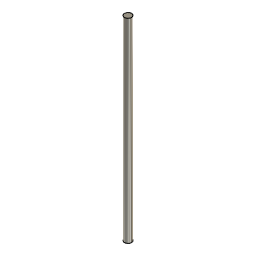
Base_Assemble (Autodesk Fusion 360 archive; units mm, degrees)
design "Rod"
Autodesk Fusion 360 part; units mm, degrees
(part 1 of 2)
sketch "Sketch1" plane through (0, 0, 0) normal (0, 0, 1) x (1, 0, 0)
  circle A0 centre (0, 0) radius 2
  dimension "d1" = 4
  constraint coincident A0.centre origin
  measures "d1" diameter of A0
extrude "Extrude1" add sketch "Sketch1" along normal blind 110

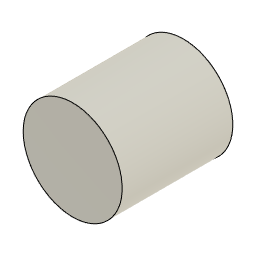
design "_Mug"
Autodesk Fusion 360 part; units mm, degrees
sketch "Sketch1" plane through (0, 0, 0) normal (0, 1, 0) x (1, 0, 0)
  circle A0 centre (0, 0) radius 42.5
  dimension "d1" = 85
  constraint coincident A0.centre origin
  measures "d1" diameter of A0
extrude "Extrude1" add sketch "Sketch1" against normal blind 95

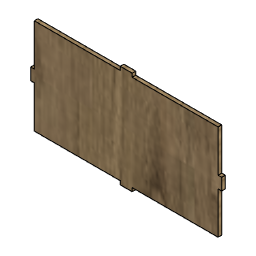
design "LongWall_"
Autodesk Fusion 360 part; units mm, degrees
sketch "Sketch1" plane through (0, 0, 0) normal (0, 1, 0) x (1, 0, 0)
  line L0 (117, 83.2352) -> (40, 83.2352)
  line L1 (40, 83.2352) -> (45, 83.2352)
  line L2 (40, 83.2352) -> (40, 43.2352)
  line L3 (40, 3.2352) -> (45, 3.2352)
  line L4 (117, 43.2352) -> (117, 83.2352)
  line L5 (117, 38.2352) -> (117, 43.2352)
  line L6 (45, 83.2352) -> (45, 86.2352)
  line L7 (120, 83.4704) -> (45, 83.4704)
  line L8 (-37, 83.2352) -> (40, 83.2352)
  line L9 (-37, 3.2352) -> (40, 3.2352)
  line L10 (40, 43.2352) -> (-37, 43.2352)
  line L11 (40, 43.2352) -> (117, 43.2352)
  line L12 (117, 3.2352) -> (40, 3.2352)
  line L13 (45, 0.2352) -> (40, 0.2352)
  line L14 (40, 86.2352) -> (40, 83.2352)
  line L15 (40, 83.2352) -> (40, 43.2352)
  line L16 (117, 43.2352) -> (117, 3.2352)
  line L17 (45, 86.4704) -> (120, 86.4704)
  line L18 (45, 0) -> (120, 0)
  line L19 (120, 48.2352) -> (117, 48.2352)
  line L20 (117, 43.2352) -> (120, 43.2352)
  line L21 (45, 3.2352) -> (45, 0.2352)
  line L22 (120, 43.2352) -> (120, 48.2352)
  line L23 (45, 86.2352) -> (40, 86.2352)
  line L24 (40, 86.2352) -> (40, 83.2352)
  line L25 (120, 0) -> (120, 3)
  line L26 (117, 43.2352) -> (120, 43.2352)
  line L27 (120, 38.2352) -> (117, 38.2352)
  line L28 (40, 43.2352) -> (117, 43.2352)
  line L29 (120, 43.2352) -> (120, 38.2352)
  line L30 (40, 43.2352) -> (-37, 43.2352)
  line L31 (40, 3.2352) -> (40, 43.2352)
  line L32 (117, 48.2352) -> (117, 43.2352)
  line L33 (45, 83.4704) -> (45, 86.4704)
  line L34 (120, 86.4704) -> (120, 83.4704)
  line L35 (45, 3) -> (45, 0)
  line L36 (-40, 48.2352) -> (-37, 48.2352)
  line L37 (-40, 38.2352) -> (-37, 38.2352)
  line L38 (35, 83.2352) -> (35, 86.2352)
  line L39 (40, 3.2352) -> (40, 43.2352)
  line L40 (-40, 43.2352) -> (-40, 48.2352)
  line L41 (40, 0.2352) -> (40, 3.2352)
  line L42 (-40, 43.2352) -> (-40, 38.2352)
  line L43 (35, 83.4704) -> (35, 86.4704)
  line L44 (35, 3.2352) -> (35, 0.2352)
  line L45 (35, 86.4704) -> (-40, 86.4704)
  line L46 (-37, 38.2352) -> (-37, 43.2352)
  line L47 (-37, 43.2352) -> (-37, 3.2352)
  line L48 (40, 3.2352) -> (35, 3.2352)
  line L49 (-37, 43.2352) -> (-37, 83.2352)
  line L50 (120, 3) -> (45, 3)
  line L51 (-40, 83.4704) -> (35, 83.4704)
  line L52 (35, 86.2352) -> (40, 86.2352)
  line L53 (40, 83.2352) -> (35, 83.2352)
  line L54 (-37, 43.2352) -> (-40, 43.2352)
  line L55 (40, 0.2352) -> (40, 3.2352)
  line L56 (-37, 48.2352) -> (-37, 43.2352)
  line L57 (35, 0.2352) -> (40, 0.2352)
  line L58 (-40, 3) -> (35, 3)
  line L59 (-37, 43.2352) -> (-40, 43.2352)
  line L60 (35, 0) -> (-40, 0)
  line L61 (35, 3) -> (35, 0)
  point P0 (0, 86.4704)
  point P1 (80, 86.4704)
  point P2 (80, 0)
  dimension "d1" = 77
  dimension "d2" = 40
  dimension "d3" = 5
  dimension "d4" = 3
  dimension "d5" = 3
  dimension "d6" = 5
  constraint horizontal L9
  constraint vertical L39
  constraint horizontal L10
  constraint vertical L47
  constraint horizontal L48
  constraint vertical L44
  constraint horizontal L57
  constraint vertical L41
  constraint vertical L42
  constraint perpendicular L42 L59
  constraint horizontal L37
  constraint parallel L42 L46
  constraint symmetric P2 origin L39
  constraint symmetric L60.start L18.start L39
  constraint symmetric L60.end L18.end L39
  constraint symmetric L58.start L25.end L39
  constraint symmetric L58.end L35.start L39
  constraint symmetric L9.start L12.start L39
  constraint symmetric L3.start L9.end L39
  constraint symmetric L2.end L10.start L39
  constraint symmetric L4.start L10.end L39
  constraint symmetric L3.end L44.start L39
  constraint symmetric L13.start L44.end L39
  constraint symmetric L13.end L41.start L39
  constraint symmetric L20.end L40.start L39
  constraint symmetric L27.start L37.start L39
  constraint symmetric L5.start L37.end L39
  constraint symmetric P0 origin L28
  constraint symmetric L17.start L18.start L28
  constraint symmetric L17.end L18.end L28
  constraint symmetric L7.start L25.end L28
  constraint symmetric L7.end L35.start L28
  constraint symmetric L9.start L8.start L28
  constraint symmetric L3.start L0.end L28
  constraint symmetric L2.end L10.start L28
  constraint symmetric L10.end L30.end L28
  constraint symmetric L44.start L38.start L28
  constraint symmetric L44.end L38.end L28
  constraint symmetric L13.end L14.start L28
  constraint symmetric L40.start L42.start L28
  constraint symmetric L37.start L36.start L28
  constraint symmetric L37.end L36.end L28
  constraint symmetric L20.end L22.start L28
  constraint symmetric L3.end L1.end L28
  constraint symmetric L5.start L19.end L28
  constraint symmetric L13.start L6.end L28
  constraint symmetric L27.start L19.start L28
  constraint symmetric L4.start L5.end L28
  constraint symmetric L0.end L3.start L28
  constraint symmetric L0.start L12.start L28
  constraint symmetric L43.start L58.end L28
  constraint symmetric L43.end L60.start L28
  constraint symmetric P1 P2 L28
  constraint symmetric L51.start L58.start L28
  constraint symmetric L45.end L60.end L28
  measures "d1" distance of L3.start L9.start
  measures "d2" distance of L10.end L9.start
  measures "d3" distance of L44.start L3.start
  measures "d4" distance of L13.end L3.start
  measures "d5" distance of L10.end L40.start
  measures "d6" distance of L10.end L37.end
extrude "Extrude1" add sketch "Sketch1" along normal blind 3 contours L0 L1 L2 L4 L11 L15 L28 L32 | L0 L1 L6 L14 L23 L24 L33 | L4 L19 L20 L22 L26 L32 | L2 L8 L10 L15 L30 L49 L53 L56 | L8 L14 L24 L38 L43 L52 L53 | L5 L16 L20 L26 L27 L29 | L3 L5 L11 L12 L16 L28 L31 L39 | L9 L10 L30 L31 L39 L46 L47 L48 | L36 L40 L49 L54 L56 L59 | L37 L42 L46 L47 L54 L59 | L9 L41 L44 L48 L55 L57 L61 | L3 L12 L13 L21 L35 L41 L55
ref_plane "WorkPlane1" through (40, 0, -43.2352) normal (0, -1, 0) x (-1, 0, 0)
sketch "Sketch2" plane through (0, 0, 0) normal (0, -1, 0) x (-1, 0, 0)
  line L0 (40, 3.2352) -> (45, 3.2352)
  line L1 (117, 48.2352) -> (117, 43.2352)
  line L2 (35, 83.4704) -> (35, 86.4704)
  line L3 (-37, 43.2352) -> (-37, 83.2352)
  line L4 (120, 48.2352) -> (117, 48.2352)
  line L5 (-37, 43.2352) -> (-37, 3.2352)
  line L6 (-37, 48.2352) -> (-37, 43.2352)
  line L7 (35, 83.2352) -> (35, 86.2352)
  line L8 (35, 3.2352) -> (35, 0.2352)
  line L9 (-40, 48.2352) -> (-37, 48.2352)
  line L10 (35, 3) -> (35, 0)
  line L11 (45, 83.4704) -> (45, 86.4704)
  line L12 (-40, 43.2352) -> (-40, 38.2352)
  line L13 (-40, 3) -> (35, 3)
  line L14 (117, 83.2352) -> (40, 83.2352)
  line L15 (35, 86.2352) -> (40, 86.2352)
  line L16 (117, 3.2352) -> (40, 3.2352)
  line L17 (40, 3.2352) -> (35, 3.2352)
  line L18 (35, 0.2352) -> (40, 0.2352)
  line L19 (-37, 83.2352) -> (40, 83.2352)
  line L20 (40, 83.2352) -> (45, 83.2352)
  line L21 (45, 0.2352) -> (40, 0.2352)
  line L22 (45, 86.2352) -> (40, 86.2352)
  line L23 (120, 43.2352) -> (120, 38.2352)
  line L24 (120, 38.2352) -> (117, 38.2352)
  line L25 (117, 43.2352) -> (117, 83.2352)
  line L26 (-37, 3.2352) -> (40, 3.2352)
  line L27 (-40, 43.2352) -> (-40, 48.2352)
  line L28 (120, 86.4704) -> (120, 83.4704)
  line L29 (45, 83.2352) -> (45, 86.2352)
  line L30 (117, 43.2352) -> (117, 3.2352)
  line L31 (45, 3) -> (45, 0)
  line L32 (45, 3.2352) -> (45, 0.2352)
  line L33 (120, 43.2352) -> (120, 48.2352)
  line L34 (-40, 38.2352) -> (-37, 38.2352)
  line L35 (117, 38.2352) -> (117, 43.2352)
  point P0 (0, 86.4704)
  point P1 (80, 86.4704)
  point P2 (80, 0)
  dimension "d10" = 77
  dimension "d11" = 40
  dimension "d12" = 5
  dimension "d13" = 3
  dimension "d14" = 3
  dimension "d15" = 5
  constraint horizontal L26
  constraint vertical L5
  constraint horizontal L17
  constraint vertical L8
  constraint horizontal L18
  constraint vertical L12
  constraint horizontal L34
  measures "d10" distance of L0.start L5.end
  measures "d11" distance of L3.start L5.end
  measures "d12" distance of L8.start L0.start
  measures "d13" distance of L18.end L0.start
  measures "d14" distance of L12.start L3.start
  measures "d15" distance of L3.start L34.end

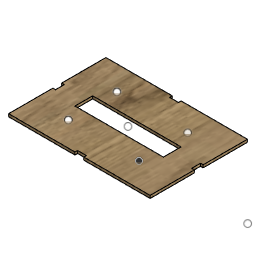
design "Roof"
Autodesk Fusion 360 part; units mm, degrees
sketch "Sketch1" plane through (0, 0, 0) normal (0, 0, 1) x (1, 0, 0)
  line L0 (-162.8452, 27.5) -> (-242.8452, 82.5) construction
  line L1 (-242.8452, 27.5) -> (-239.8452, 27.5)
  line L2 (-162.8452, 82.5) -> (-242.8452, 82.5)
  line L3 (-242.8452, 27.5) -> (-162.8452, 82.5) construction
  line L4 (-112.8452, 37.5) -> (-212.8452, 37.5)
  line L5 (-167.8452, 82.5) -> (-167.8452, 79.5)
  line L6 (-82.8452, 27.5) -> (-162.8452, -27.5) construction
  line L7 (-82.8452, 22.5) -> (-82.8452, 27.5)
  line L8 (-162.8452, 27.5) -> (-242.8452, -27.5) construction
  line L9 (-162.8452, 27.5) -> (-82.8452, -27.5) construction
  line L10 (-112.8452, 17.5) -> (-112.8452, 37.5)
  line L11 (-162.8452, 82.5) -> (-82.8452, 82.5)
  line L12 (-162.8452, 27.5) -> (-82.8452, 82.5) construction
  line L13 (-162.8452, 27.5) -> (-162.8452, -27.5)
  line L14 (-157.8452, -27.5) -> (-157.8452, -24.5)
  line L15 (-157.8452, 82.5) -> (-157.8452, 79.5)
  line L16 (-242.8452, 27.5) -> (-162.8452, -27.5) construction
  line L17 (-85.8452, 22.5) -> (-82.8452, 22.5)
  line L18 (-157.8452, -24.5) -> (-162.8452, -24.5)
  line L19 (-85.8452, 27.5) -> (-85.8452, 22.5)
  line L20 (-162.8452, 82.5) -> (-157.8452, 82.5)
  line L21 (-82.8452, 27.5) -> (-85.8452, 27.5)
  line L22 (-157.8452, 79.5) -> (-162.8452, 79.5)
  line L23 (-162.8452, -24.5) -> (-162.8452, -27.5)
  line L24 (-242.8452, 82.5) -> (-242.8452, 27.5)
  line L25 (-239.8452, 32.5) -> (-242.8452, 32.5)
  line L26 (-162.8452, -27.5) -> (-167.8452, -27.5)
  line L27 (-167.8452, 79.5) -> (-162.8452, 79.5)
  line L28 (-239.8452, 27.5) -> (-239.8452, 22.5)
  line L29 (-239.8452, 27.5) -> (-239.8452, 32.5)
  line L30 (-162.8452, 27.5) -> (-162.8452, 82.5)
  line L31 (-242.8452, 27.5) -> (-239.8452, 27.5)
  line L32 (-162.8452, 27.5) -> (-162.8452, -27.5)
  line L33 (-167.8452, -27.5) -> (-167.8452, -24.5)
  line L34 (-239.8452, 22.5) -> (-242.8452, 22.5)
  line L35 (-82.8452, 32.5) -> (-82.8452, 27.5)
  line L36 (-85.8452, 32.5) -> (-82.8452, 32.5)
  line L37 (-242.8452, 27.5) -> (-162.8452, 27.5)
  line L38 (-242.8452, 27.5) -> (-162.8452, 27.5)
  line L39 (-82.8452, 27.5) -> (-162.8452, 27.5)
  line L40 (-112.8452, 17.5) -> (-212.8452, 37.5) construction
  line L41 (-82.8452, 27.5) -> (-162.8452, 27.5)
  line L42 (-82.8452, 27.5) -> (-162.8452, 82.5) construction
  line L43 (-212.8452, 17.5) -> (-112.8452, 17.5)
  line L44 (-162.8452, 82.5) -> (-167.8452, 82.5)
  line L45 (-167.8452, -24.5) -> (-162.8452, -24.5)
  line L46 (-242.8452, 22.5) -> (-242.8452, 27.5)
  line L47 (-162.8452, 79.5) -> (-162.8452, 82.5)
  line L48 (-162.8452, 27.5) -> (-162.8452, 82.5)
  line L49 (-242.8452, 32.5) -> (-242.8452, 27.5)
  line L50 (-242.8452, -27.5) -> (-242.8452, 27.5)
  line L51 (-212.8452, 37.5) -> (-212.8452, 17.5)
  line L52 (-162.8452, -24.5) -> (-162.8452, -27.5)
  line L53 (-212.8452, 17.5) -> (-112.8452, 37.5) construction
  line L54 (-82.8452, -27.5) -> (-82.8452, 27.5)
  line L55 (-162.8452, -27.5) -> (-242.8452, -27.5)
  line L56 (-162.8452, -27.5) -> (-157.8452, -27.5)
  line L57 (-162.8452, -27.5) -> (-82.8452, -27.5)
  line L58 (-82.8452, 27.5) -> (-85.8452, 27.5)
  line L59 (-162.8452, 79.5) -> (-162.8452, 82.5)
  line L60 (-82.8452, 82.5) -> (-82.8452, 27.5)
  line L61 (-85.8452, 27.5) -> (-85.8452, 32.5)
  point P0 (-162.8452, 27.5)
  point P1 (-202.8452, 0)
  point P2 (-202.8452, 0)
  point P3 (-202.8452, 55)
  point P4 (-122.8452, 0)
  point P5 (-122.8452, 55)
  point P6 (-122.8452, 55)
  point P7 (-202.8452, 55)
  point P8 (-122.8452, 0)
  dimension "d1" = 80
  dimension "d2" = 55
  dimension "d3" = 5
  dimension "d4" = 3
  dimension "d5" = 3
  dimension "d6" = 5
  dimension "d7" = 100
  dimension "d8" = 20
  constraint horizontal L41
  constraint perpendicular L32 L41
  constraint parallel L41 L57
  constraint parallel L32 L54
  constraint coincident P8 L6
  constraint coincident P8 L9
  constraint coincident P8 P4
  constraint horizontal L56
  constraint vertical L14
  constraint horizontal L18
  constraint vertical L23
  constraint horizontal L58
  constraint vertical L19
  constraint horizontal L17
  constraint vertical L7
  constraint symmetric P2 P8 L32
  constraint symmetric L1.start L6.start L32
  constraint symmetric P0 L0.start L32
  constraint symmetric L6.end L13.end L32
  constraint symmetric L8.end L9.end L32
  constraint symmetric L26.end L14.start L32
  constraint symmetric L14.end L33.end L32
  constraint symmetric L18.end L23.start L32
  constraint symmetric L19.start L1.end L32
  constraint symmetric L17.start L28.end L32
  constraint symmetric L34.end L7.start L32
  constraint symmetric P8 P6 L41
  constraint symmetric L6.start L7.end L41
  constraint symmetric P0 L0.start L41
  constraint symmetric L2.start L6.end L41
  constraint symmetric L9.end L11.end L41
  constraint symmetric P6 P8 L41
  constraint symmetric L14.start L15.start L41
  constraint symmetric L14.end L15.end L41
  constraint symmetric L22.end L18.end L41
  constraint symmetric L19.start L21.end L41
  constraint symmetric L17.start L36.start L41
  constraint symmetric L35.start L7.start L41
  constraint symmetric L1.end L28.start L41
  constraint symmetric L5.start L26.end L41
  constraint symmetric L33.end L5.end L41
  constraint symmetric L25.start L28.end L41
  constraint symmetric L8.end L0.end L41
  constraint symmetric L1.start L3.start L41
  constraint symmetric L34.end L25.end L41
  constraint symmetric P2 P7 L41
  constraint horizontal L43
  constraint perpendicular L10 L43
  constraint parallel L4 L43
  constraint parallel L10 L51
  constraint coincident P0 L53
  constraint coincident P0 L40
  constraint coincident P0 L0.start
  measures "d1" distance of L9.end L6.end
  measures "d2" distance of P0 L6.end
  measures "d3" distance of L14.start L6.end
  measures "d4" distance of L18.end L6.end
  measures "d5" distance of L19.start L6.start
  measures "d6" distance of L7.start L6.start
  measures "d7" distance of L4.start L4.end
  measures "d8" distance of L10.start L4.start
extrude "Extrude1" add sketch "Sketch1" along normal blind 3 contours L13 L28 L32 L33 L34 L37 L38 L43 L45 L50 L51 L55 | L2 L4 L5 L24 L25 L27 L29 L30 L37 L38 L48 L51 | L10 L13 L14 L17 L18 L19 L32 L39 L41 L43 L54 L57 | L4 L10 L11 L15 L22 L30 L36 L39 L41 L48 L60 L61
ref_plane "WorkPlane1" through (-162.8452, 27.5, 3) normal (0, 0, 1) x (1, 0, 0)
sketch "Sketch2" plane through (0, 0, 3) normal (0, 0, 1) x (1, 0, 0)
  point P0 (-122.8452, 0)
  point P1 (-122.8452, 0)
  point P2 (-202.8452, 55)
  point P3 (-202.8452, 55)
  point P4 (-122.8452, 55)
  point P5 (-202.8452, 0)
  point P6 (-202.8452, 0)
  point P7 (-162.8452, 27.5)
  constraint coincident P0 P1

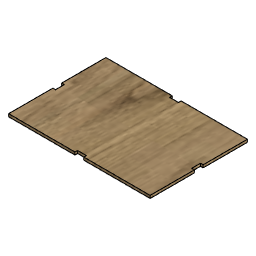
design "Floor"
Autodesk Fusion 360 part; units mm, degrees
sketch "Sketch1" plane through (0, 0, 0) normal (0, 0, 1) x (1, 0, 0)
  line L0 (-120, 27.5) -> (-40, 82.5) construction
  line L1 (-40, 27.5) -> (-120, -27.5) construction
  line L2 (-120, 27.5) -> (-117, 27.5)
  line L3 (-120, 27.5) -> (-117, 27.5)
  line L4 (-117, 22.5) -> (-120, 22.5)
  line L5 (-45, -24.5) -> (-40, -24.5)
  line L6 (-40, 27.5) -> (-120, 82.5) construction
  line L7 (-120, 27.5) -> (-40, 27.5)
  line L8 (-120, 27.5) -> (-40, 27.5)
  line L9 (-40, 82.5) -> (-45, 82.5)
  line L10 (-117, 27.5) -> (-117, 22.5)
  line L11 (-45, 82.5) -> (-45, 79.5)
  line L12 (-120, -27.5) -> (-120, 27.5)
  line L13 (-40, -27.5) -> (-120, -27.5)
  line L14 (-120, 22.5) -> (-120, 27.5)
  line L15 (40, 27.5) -> (-40, 27.5)
  line L16 (40, 27.5) -> (-40, 27.5)
  line L17 (-117, 32.5) -> (-120, 32.5)
  line L18 (-40, 82.5) -> (-120, 82.5)
  line L19 (-45, -27.5) -> (-45, -24.5)
  line L20 (-40, -27.5) -> (-45, -27.5)
  line L21 (-40, -27.5) -> (40, -27.5)
  line L22 (37, 22.5) -> (40, 22.5)
  line L23 (40, 27.5) -> (-40, -27.5) construction
  line L24 (40, 32.5) -> (40, 27.5)
  line L25 (-40, 27.5) -> (40, -27.5) construction
  line L26 (-35, 82.5) -> (-35, 79.5)
  line L27 (-35, -27.5) -> (-35, -24.5)
  line L28 (-40, 27.5) -> (-40, 82.5)
  line L29 (40, 27.5) -> (37, 27.5)
  line L30 (-35, -24.5) -> (-40, -24.5)
  line L31 (37, 27.5) -> (37, 32.5)
  line L32 (37, 32.5) -> (40, 32.5)
  line L33 (-40, 82.5) -> (40, 82.5)
  line L34 (40, 82.5) -> (40, 27.5)
  line L35 (-40, -27.5) -> (-35, -27.5)
  line L36 (40, -27.5) -> (40, 27.5)
  line L37 (-40, 82.5) -> (-35, 82.5)
  line L38 (40, 27.5) -> (-40, 82.5) construction
  line L39 (-35, 79.5) -> (-40, 79.5)
  line L40 (40, 27.5) -> (37, 27.5)
  line L41 (-40, 27.5) -> (40, 82.5) construction
  line L42 (-40, -24.5) -> (-40, -27.5)
  line L43 (-40, 27.5) -> (-40, 82.5)
  line L44 (-40, 79.5) -> (-40, 82.5)
  line L45 (40, 22.5) -> (40, 27.5)
  line L46 (-40, 27.5) -> (-40, -27.5)
  line L47 (37, 27.5) -> (37, 22.5)
  line L48 (-40, 27.5) -> (-40, -27.5)
  line L49 (-40, 79.5) -> (-40, 82.5)
  line L50 (-40, -24.5) -> (-40, -27.5)
  line L51 (-120, 27.5) -> (-40, -27.5) construction
  line L52 (-120, 32.5) -> (-120, 27.5)
  line L53 (-117, 27.5) -> (-117, 32.5)
  line L54 (-120, 82.5) -> (-120, 27.5)
  line L55 (-45, 79.5) -> (-40, 79.5)
  point P0 (-80, 55)
  point P1 (0, 55)
  point P2 (-80, 55)
  point P3 (0, 55)
  point P4 (-80, 0)
  point P5 (-80, 0)
  dimension "d1" = 80
  dimension "d2" = 55
  dimension "d3" = 5
  dimension "d4" = 3
  dimension "d5" = 3
  dimension "d6" = 5
  constraint horizontal L15
  constraint perpendicular L15 L48
  constraint parallel L15 L21
  constraint parallel L36 L48
  constraint coincident origin L23
  constraint coincident origin L25
  constraint horizontal L35
  constraint vertical L27
  constraint horizontal L30
  constraint vertical L50
  constraint horizontal L40
  constraint vertical L47
  constraint horizontal L22
  constraint vertical L45
  constraint symmetric origin P5 L48
  constraint symmetric L15.start L0.start L48
  constraint symmetric L1.start L6.start L48
  constraint symmetric L13.start L20.start L48
  constraint symmetric L21.end L1.end L48
  constraint symmetric L27.start L19.start L48
  constraint symmetric L27.end L5.start L48
  constraint symmetric L5.end L30.end L48
  constraint symmetric L2.end L29.end L48
  constraint symmetric L4.start L22.start L48
  constraint symmetric L22.end L4.end L48
  constraint symmetric P3 origin L15
  constraint symmetric L16.start L23.start L15
  constraint symmetric L1.start L6.start L15
  constraint symmetric L13.start L0.end L15
  constraint symmetric L21.end L33.end L15
  constraint symmetric origin P3 L15
  constraint symmetric L27.start L26.start L15
  constraint symmetric L27.end L26.end L15
  constraint symmetric L5.end L39.end L15
  constraint symmetric L29.end L31.start L15
  constraint symmetric L31.end L22.start L15
  constraint symmetric L24.start L22.end L15
  constraint symmetric L2.end L3.end L15
  constraint symmetric L19.start L9.end L15
  constraint symmetric L5.start L11.end L15
  constraint symmetric L4.start L17.start L15
  constraint symmetric L1.end L6.end L15
  constraint symmetric L0.start L2.start L15
  constraint symmetric L17.end L4.end L15
  constraint symmetric P2 P5 L15
  measures "d1" distance of L13.start L21.end
  measures "d2" distance of L1.start L13.start
  measures "d3" distance of L27.start L13.start
  measures "d4" distance of L5.end L13.start
  measures "d5" distance of L15.start L29.end
  measures "d6" distance of L15.start L22.end
extrude "Extrude1" add sketch "Sketch1" along normal blind 3 contours L7 L8 L11 L17 L18 L28 L43 L53 L54 L55 | L4 L5 L7 L8 L10 L12 L13 L19 L46 L48 | L15 L16 L26 L28 L31 L32 L33 L34 L39 L43 | L15 L16 L21 L22 L27 L30 L36 L46 L47 L48
ref_plane "WorkPlane1" through (-40, 27.5, 3) normal (0, 0, 1) x (1, 0, 0)
sketch "Sketch2" plane through (0, 0, 0) normal (0, 0, 1) x (1, 0, 0)
  line L0 (-35, 79.5) -> (-40, 79.5)
  line L1 (-40, -27.5) -> (40, -27.5)
  line L2 (-40, 79.5) -> (-40, 82.5)
  line L3 (40, 27.5) -> (37, 27.5)
  line L4 (-45, 79.5) -> (-40, 79.5)
  line L5 (-40, 82.5) -> (-45, 82.5)
  line L6 (-35, -27.5) -> (-35, -24.5)
  line L7 (-40, 82.5) -> (-35, 82.5)
  line L8 (40, -27.5) -> (40, 27.5)
  line L9 (40, 27.5) -> (37, 27.5)
  line L10 (-40, 82.5) -> (40, 82.5)
  line L11 (-35, 82.5) -> (-35, 79.5)
  line L12 (-40, -27.5) -> (-45, -27.5)
  line L13 (40, 82.5) -> (40, 27.5)
  line L14 (37, 27.5) -> (37, 22.5)
  line L15 (37, 22.5) -> (40, 22.5)
  line L16 (-40, -27.5) -> (-120, -27.5)
  line L17 (37, 32.5) -> (40, 32.5)
  line L18 (-120, 82.5) -> (-120, 27.5)
  line L19 (-117, 27.5) -> (-117, 22.5)
  line L20 (-35, -24.5) -> (-40, -24.5)
  line L21 (-120, 32.5) -> (-120, 27.5)
  line L22 (-117, 27.5) -> (-117, 32.5)
  line L23 (-120, 27.5) -> (-117, 27.5)
  line L24 (-45, -27.5) -> (-45, -24.5)
  line L25 (-120, 22.5) -> (-120, 27.5)
  line L26 (-117, 32.5) -> (-120, 32.5)
  line L27 (-120, -27.5) -> (-120, 27.5)
  line L28 (-45, 82.5) -> (-45, 79.5)
  line L29 (-120, 27.5) -> (-117, 27.5)
  line L30 (-117, 22.5) -> (-120, 22.5)
  line L31 (-40, 79.5) -> (-40, 82.5)
  line L32 (40, 22.5) -> (40, 27.5)
  line L33 (-40, 82.5) -> (-120, 82.5)
  line L34 (-45, -24.5) -> (-40, -24.5)
  line L35 (40, 32.5) -> (40, 27.5)
  line L36 (37, 27.5) -> (37, 32.5)
  point P0 (-80, 0)
  point P1 (-80, 0)
  point P2 (-80, 55)
  point P3 (-80, 55)
  point P4 (0, 55)
  point P5 (0, 55)
  dimension "d11" = 80
  dimension "d13" = 5
  dimension "d14" = 3
  dimension "d15" = 3
  dimension "d16" = 5
  constraint vertical L6
  constraint horizontal L20
  constraint horizontal L9
  constraint vertical L14
  constraint horizontal L15
  constraint vertical L32
  measures "d11" distance of L1.start L1.end
  measures "d13" distance of L1.start L6.start
  measures "d14" distance of L1.start L20.end
  measures "d15" distance of L3.end L3.start
  measures "d16" distance of L3.start L15.end

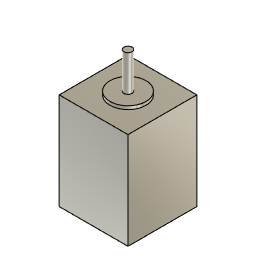
design "_StepperMotor"
Autodesk Fusion 360 part; units mm, degrees
sketch "Sketch2" plane through (0, 0, 0) normal (0, 0, 1) x (1, 0, 0)
  line L0 (0, 0) -> (42, 0)
  line L1 (42, 0) -> (42, 42)
  line L2 (42, 42) -> (0, 42)
  line L3 (0, 42) -> (0, 0)
  dimension "d1" = 42
  dimension "d2" = 42
  constraint horizontal L0
  constraint vertical L1
  constraint horizontal L2
  constraint vertical L3
  constraint coincident L0.start L3.end
  measures "d1" distance of L0.start L2.end
  measures "d2" distance of L0.start L0.end
extrude "Extrude1" add sketch "Sketch2" along normal blind 59
sketch "Sketch3" plane through (0, 0, 59) normal (0, 0, 1) x (-1, 0, 0)
  line L0 (0, -42) -> (0, 0)
  line L1 (0, 0) -> (-42, 0)
  line L2 (-42, 0) -> (-42, -42)
  line L3 (-42, -42) -> (0, -42)
  line L4 (0, -42) -> (-42, 0) construction
  line L5 (-42, -42) -> (0, 0) construction
  circle A0 centre (-21, -21) radius 11
  circle A1 centre (-21, -21) radius 2.5
  line L6 (-21, -55) -> (-21, 14) construction
  line L7 (-4, -49.5981) -> (-4, 7) construction
  line L8 (6.5, -21) -> (-54.5, -21) construction
  line L9 (6.5, -37.5) -> (-46.0507, -37.5) construction
  circle A2 centre (-5.5, -36) radius 1.5
  circle A3 centre (-36.5, -36) radius 1.5
  dimension "d5" = 22
  dimension "d9" = 5
  dimension "d15" = 21
  dimension "d16" = 17
  dimension "d17" = 21
  dimension "d18" = 16.5
  dimension "d19" = 1.5
  constraint coincident L0.start L3.end
  constraint coincident L1.end L2.start
  constraint coincident L2.end L3.start
  constraint coincident L0.end L1.start
  constraint midpoint L5 A0.centre
  constraint concentric A0 A1
  constraint perpendicular L3 L6
  constraint vertical L7
  constraint horizontal L8
  constraint horizontal L9
  constraint tangent L7 A2
  constraint tangent L9 A2
  constraint symmetric L6 A2 A3
  measures "d5" diameter of A0
  measures "d9" diameter of A1
  measures "d15" distance of L0 L6
  measures "d16" distance of L6 L7
  measures "d17" distance of L3 L8
  measures "d18" distance of L8 L9
  measures "d19" radius of A2
extrude "Extrude3" add sketch "Sketch3" along normal blind 24 contours A1
extrude "Extrude4" add sketch "Sketch3" along normal blind 2 contours A0
equation "d10 = 22 mm + 2 mm"
equation "d15 = ( 42 / 2 ) * 1 mm"
equation "d16 = ( 34 / 2 ) * 1 mm"
equation "d17 = ( 42 / 2 ) * 1 mm"
equation "d18 = ( 33 / 2 ) * 1 mm"
equation "d19 = ( 3 / 2 ) * 1 mm"

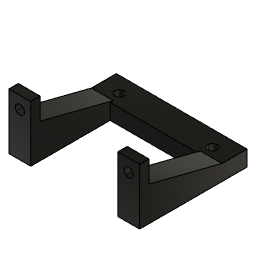
design "_stepper_motor_fixer"
Autodesk Fusion 360 part; units mm, degrees
sketch "Sketch1" plane through (0, 0, 0) normal (0, 0, 1) x (1, 0, 0)
  circle A0 centre (-5.5, -36) radius 1.5
  circle A1 centre (-36.5, -36) radius 1.5
  line L0 (0, 0) -> (42, 0)
  line L1 (42, 0) -> (42, 8)
  line L2 (42, 8) -> (0, 8)
  line L3 (0, 8) -> (0, 0)
  line L4 (21, 12) -> (21, -11) construction
  line L5 (4.5, 10) -> (4.5, -10) construction
  line L6 (-3, 1.5) -> (48, 1.5) construction
  circle A2 centre (6, 3) radius 1.5
  circle A3 centre (36, 3) radius 1.5
  dimension "d1" = 1.5
  dimension "d2" = 42
  dimension "d3" = 8
  dimension "d4" = 21
  dimension "d5" = 4.5
  dimension "d6" = 51
  dimension "d7" = 6.5
  dimension "d8" = 1.5
  constraint horizontal L0
  constraint vertical L1
  constraint horizontal L2
  constraint vertical L3
  constraint coincident L0.start L3.end
  constraint vertical L4
  constraint perpendicular L2 L5
  constraint horizontal L6
  constraint tangent L5 A2
  constraint tangent L6 A2
  constraint symmetric L4 A2 A3
  measures "d1" radius of A0
  measures "d2" distance of L0.start L0.end
  measures "d3" distance of L0.end L1.end
  measures "d4" distance of L3 L4
  measures "d5" distance of L3 L5
  measures "d6" distance of L6.start L6.end
  measures "d7" distance of L2 L6
  measures "d8" radius of A2
extrude "Extrude1" add sketch "Sketch1" along normal blind 5 contours L0 L1 L2 L3
sketch "Sketch2" plane through (0, 0, 5) normal (0, 0, 1) x (-1, 0, 0)
  circle A0 centre (-6, -3) radius 1.5
  circle A1 centre (-36, -3) radius 1.5
  line L0 (0, -8) -> (0, 0)
  line L1 (0, 0) -> (-42, 0)
  line L2 (-42, 0) -> (-42, -8)
  line L3 (-42, -8) -> (0, -8)
  line L4 (0, 26.5) -> (-42, 26.5) construction
  line L5 (-42, 26.5) -> (-32, 26.5) construction
  line L6 (-7, -10) -> (-7, 37) construction
  line L7 (0, 0) -> (0, 26.5)
  line L8 (-7, 26.5) -> (-7, 0)
  line L9 (0, 26.5) -> (-7, 26.5)
  line L10 (-21, -11) -> (-21, 34) construction
  line L11 (-42, 0) -> (-42, 26.5)
  line L12 (-35, 26.5) -> (-35, 0)
  line L13 (-42, 26.5) -> (-35, 26.5)
  dimension "d11" = 34.5
  dimension "d12" = 7
  dimension "d13" = 21
  constraint horizontal L4
  constraint coincident L4 L5.end
  constraint vertical L6
  constraint coincident L0.end L1.start
  constraint perpendicular L4 L7
  constraint coincident L4 L8.start
  constraint coincident L6 L8.start
  constraint coincident L1 L8.end
  constraint coincident L6 L8.end
  constraint perpendicular L4 L10
  constraint symmetric L4.start L10 L4.end
  constraint symmetric L0.end L10 L1.end
  constraint symmetric L8.start L10 L12.start
  constraint symmetric L8.end L10 L12.end
  measures "d11" distance of L3 L4
  measures "d12" distance of L0 L6
  measures "d13" distance of L0 L10
extrude "Extrude2" add sketch "Sketch2" against normal blind 5 contours L1 L7 L8 L9 | L1 L11 L12 L13
sketch "Sketch3" plane through (0, -26.5, 0) normal (0, -1, 0) x (1, 0, 0)
  line L0 (7, 5) -> (0, 5)
  line L1 (0, 5) -> (0, 0)
  line L2 (0, 0) -> (7, 0)
  line L3 (7, 0) -> (7, 5)
  line L4 (21, -4) -> (21, 21) construction
  line L5 (7, 5) -> (0, 5)
  line L6 (0, 5) -> (0, 18)
  line L7 (0, 18) -> (7, 18)
  line L8 (7, 18) -> (7, 5)
  line L9 (-1, 14) -> (10.5, 14) construction
  line L10 (3.5, 18.5) -> (3.5, 2.8396) construction
  circle A0 centre (3.5, 14) radius 1.5
  circle A1 centre (38.5, 14) radius 1.5
  line L11 (35, 5) -> (42, 5)
  line L12 (42, 5) -> (42, 18)
  line L13 (35, 18) -> (35, 5)
  line L14 (42, 18) -> (35, 18)
  dimension "d16" = 21
  dimension "d17" = 13
  dimension "d19" = 4
  dimension "d20" = 7
  dimension "d21" = 3.5
  dimension "d22" = 3
  constraint perpendicular L0 L4
  constraint horizontal L5
  constraint vertical L6
  constraint horizontal L7
  constraint vertical L8
  constraint coincident L0.start L3.end
  constraint horizontal L9
  constraint perpendicular L7 L10
  constraint coincident L10 A0.centre
  constraint coincident L9 A0.centre
  constraint symmetric L4 L0.start L11.start
  constraint symmetric L4 L0.end L11.end
  constraint symmetric L4 L6.end L12.end
  constraint symmetric L4 L7.end L13.start
  constraint symmetric L4 A0 A1
  measures "d16" distance of L1 L4
  measures "d17" distance of L0.end L6.end
  measures "d19" distance of L7 L9
  measures "d20" distance of L6.end L7.end
  measures "d21" distance of L6 L10
  measures "d22" diameter of A0
extrude "Extrude3" add sketch "Sketch3" against normal blind 3 contours L0 L5 L6 L7 L8 | L11 L12 L13 L14
sketch "fixer" plane through (0, 0, 0) normal (1, 0, 0) x (0, 1, 0)
  line L0 (-22, 11) -> (-29, 11) construction
  line L1 (-26.5, 18) -> (-23.5, 18)
  line L2 (0, 8) -> (0, -1.5191) construction
  line L3 (0, 5) -> (-23.5, 11)
  line L4 (0, 5) -> (-23.5, 5)
  line L5 (-23.5, 11) -> (-23.5, 5)
  dimension "d25" = 7
  constraint horizontal L0
  constraint vertical L2
  constraint coincident L2 L3.start
  constraint coincident L0 L3.end
  constraint perpendicular L2 L4
  constraint perpendicular L4 L5
  measures "d25" distance of L0 L1
extrude "Extrude5" add sketch "fixer" along normal blind 7
ref_plane "WorkPlane1" through (42, 0, 0) normal (1, 0, 0) x (0, 1, 0)
sketch "Sketch6" plane through (42, 0, 0) normal (1, 0, 0) x (0, 1, 0)
  line L0 (-26.5, 0) -> (8, 0)
  line L1 (8, 0) -> (8, 5)
  line L2 (8, 5) -> (-23.5, 5)
  line L3 (-23.5, 5) -> (-23.5, 18)
  line L4 (-23.5, 18) -> (-26.5, 18)
  line L5 (-26.5, 18) -> (-26.5, 0)
  line L6 (0, 5) -> (-23.5, 11)
  line L7 (-23.5, 11) -> (-23.5, 5)
  line L8 (0, 5) -> (-23.5, 5)
  constraint perpendicular L7 L8
extrude "Extrude6" add sketch "Sketch6" against normal blind 7 contours L2 L3 L6 L7 L8
sketch "Sketch7" plane through (0, 0, 5) normal (0, 0, 1) x (-1, 0, 0)
  circle A0 centre (-36, -3) radius 1.5
  circle A1 centre (-6, -3) radius 1.5
  line L0 (-35, 0) -> (-42, 0)
  line L1 (-42, 0) -> (-42, -8)
  line L2 (-42, -8) -> (0, -8)
  line L3 (0, -8) -> (0, 0)
  line L4 (0, 0) -> (-7, 0)
  line L5 (-7, 0) -> (-35, 0)
  line L6 (-7, 0) -> (-35, 0)
  line L7 (-35, 0) -> (-35, 1)
  line L8 (-35, 1) -> (-7, 1)
  line L9 (-7, 1) -> (-7, 0)
  dimension "d33" = 1
  constraint horizontal L6
  constraint vertical L7
  constraint horizontal L8
  constraint vertical L9
  constraint coincident L4.end L5.start
  measures "d33" distance of L0.start L7.end
extrude "Extrude7" add sketch "Sketch7" against normal blind 5 contours L5 L6 L7 L8 L9
equation "d4 = ( 42 / 2 ) * 1 mm"
equation "d8 = ( 3 / 2 ) * 1 mm"
equation "d13 = ( 42 / 2 ) * 1 mm"
equation "d16 = ( 42 / 2 ) * 1 mm"

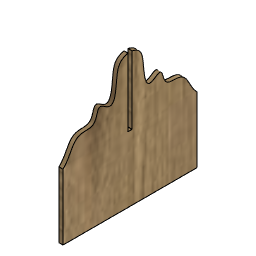
design "Base_Foot"
Autodesk Fusion 360 part; units mm, degrees
sketch "Sketch1" plane through (0, 0, 0) normal (1, 0, 0) x (0, 1, 0)
  line L0 (0, 0) -> (0, 100) construction
  spline S0 degree 5 poles (-50, 49) (-49.5004, 49.4476) (-48.5446, 50.4053) (-47.2407, 52.0292) (-45.7311, 54.5085) (-44.0522, 57.789) (-42.3664, 60.8266) (-40.4714, 63.2243) (-38.2344, 64.7235) (-35.6446, 65.308) (-32.8779, 65.334) (-30.2155, 65.3602) (-27.9429, 65.9395) (-26.2619, 67.4376) (-25.1834, 69.8088) (-24.4682, 72.4808) (-23.7735, 74.6973) (-22.7671, 75.7922) (-21.2553, 75.4915) (-19.3037, 74.2023) (-17.1367, 72.7086) (-15.0394, 71.8776) (-13.2584, 72.3576) (-11.907, 74.2934) (-10.99, 77.4724) (-10.424, 81.4506) (-10.0586, 85.6893) (-9.6963, 89.6745) (-9.1121, 93.07) (-8.0745, 95.7609) (-6.3656, 97.7647) (-4.3149, 98.8953) (-2.3351, 99.5256) (-0.8122, 99.8567) (0, 100) knots 0 0 0 0 0 0 0.033333 0.066667 0.1 0.133333 0.166667 0.2 0.233333 0.266667 0.3 0.333333 0.366667 0.4 0.433333 0.466667 0.5 0.533333 0.566667 0.6 0.633333 0.666667 0.7 0.733333 0.766667 0.8 0.833333 0.866667 0.9 0.933333 0.966667 1 1 1 1 1 1
  spline S1 degree 5 poles (50, 49) (49.5004, 49.4476) (48.5446, 50.4053) (47.2407, 52.0292) (45.7311, 54.5085) (44.0522, 57.789) (42.3664, 60.8266) (40.4714, 63.2243) (38.2344, 64.7235) (35.6446, 65.308) (32.8779, 65.334) (30.2155, 65.3602) (27.9429, 65.9395) (26.2619, 67.4376) (25.1834, 69.8088) (24.4682, 72.4808) (23.7735, 74.6973) (22.7671, 75.7922) (21.2553, 75.4915) (19.3037, 74.2023) (17.1367, 72.7086) (15.0394, 71.8776) (13.2584, 72.3576) (11.907, 74.2934) (10.99, 77.4724) (10.424, 81.4506) (10.0586, 85.6893) (9.6963, 89.6745) (9.1121, 93.07) (8.0745, 95.7609) (6.3656, 97.7647) (4.3149, 98.8953) (2.3351, 99.5256) (0.8122, 99.8567) (0, 100) knots 0 0 0 0 0 0 0.033333 0.066667 0.1 0.133333 0.166667 0.2 0.233333 0.266667 0.3 0.333333 0.366667 0.4 0.433333 0.466667 0.5 0.533333 0.566667 0.6 0.633333 0.666667 0.7 0.733333 0.766667 0.8 0.833333 0.866667 0.9 0.933333 0.966667 1 1 1 1 1 1
  line L1 (-58.5461, 41.3423) -> (-41.4539, 56.6577)
  line L2 (-14.0459, 97.5218) -> (14.0459, 102.4782)
  line L3 (58.5461, 41.3423) -> (41.4539, 56.6577)
  line L4 (14.0459, 97.5218) -> (-14.0459, 102.4782)
  line L5 (-75, 100) -> (80, 100) construction
  line L6 (-50, 49) -> (-50, 0)
  line L7 (50, 49) -> (50, 0)
  line L8 (-50, 0) -> (50, 0)
  line L9 (-50, 49) -> (50, 49) construction
  line L10 (-1.5, 49) -> (-1.5, 99.6882)
  line L11 (1.5, 49) -> (1.5, 99.6882)
  line L12 (1.5, 49) -> (-1.5, 49)
  point P0 (-37.8878, 64.6063)
  point P1 (-26.704, 67.2808)
  point P2 (-22.6571, 75.4443)
  point P3 (-15.2004, 72.2084)
  point P4 (-9.8431, 87.8254)
  point P5 (9.8431, 87.8254)
  point P6 (37.8878, 64.6063)
  point P7 (26.704, 67.2808)
  point P8 (22.6571, 75.4443)
  point P9 (15.2004, 72.2084)
  dimension "d8" = 100
  dimension "d10" = 50
  dimension "d11" = 49
  dimension "d12" = 1.5
  constraint coincident L0.start origin
  constraint midpoint L1 S0.start
  constraint midpoint L0.end L2
  constraint symmetric L0 S1.start S0.start
  constraint symmetric S0.end L0 S1.end
  constraint symmetric L0 P0 P6
  constraint symmetric L0 P1 P7
  constraint symmetric L0 P2 P8
  constraint symmetric L0 P3 P9
  constraint symmetric L0 P4 P5
  constraint symmetric L0 L1.start L3.start
  constraint symmetric L0 L1.end L3.end
  constraint symmetric L0 L2.start L4.start
  constraint symmetric L0 L2.end L4.end
  constraint horizontal L5
  constraint vertical L6
  constraint symmetric L0 S0.start S1.start
  constraint symmetric L0 L6.end L7.end
  constraint vertical L10
  constraint coincident S0 L10.end
  constraint symmetric L0 L10.start L11.start
  constraint symmetric L0 L10.end L11.end
  constraint coincident L9 L10.start
  measures "d8" distance of L0.start L0.end
  measures "d10" distance of L0 L6
  measures "d11" distance of L8 L9
  measures "d12" distance of L0 L10
extrude "Extrude2" add sketch "Sketch1" along normal blind 3 contours S0 S1 L6 L7 L8 L10 L11 L12
ref_plane "WorkPlane1" through (3, 0, 49.8441) normal (1, 0, 0) x (0, 1, 0)
sketch "laserexp" plane through (3, 0, 0) normal (1, 0, 0) x (0, 1, 0)
  spline S0 degree 5 poles (50, 49) (49.5004, 49.4476) (48.5446, 50.4053) (47.2407, 52.0292) (45.7311, 54.5085) (44.0522, 57.789) (42.3664, 60.8266) (40.4714, 63.2243) (38.2344, 64.7235) (35.6446, 65.308) (32.8779, 65.334) (30.2155, 65.3602) (27.9429, 65.9395) (26.2619, 67.4376) (25.1834, 69.8088) (24.4682, 72.4808) (23.7735, 74.6973) (22.7671, 75.7922) (21.2553, 75.4915) (19.3037, 74.2023) (17.1367, 72.7086) (15.0394, 71.8776) (13.2584, 72.3576) (11.907, 74.2934) (10.99, 77.4724) (10.424, 81.4506) (10.0586, 85.6893) (9.6963, 89.6745) (9.1121, 93.07) (8.0745, 95.7609) (6.4983, 97.6092) (4.7065, 98.6714) (3.0815, 99.2699) (1.9488, 99.5793) (1.5, 99.6882) knots 0 0 0 0 0 0 0.033333 0.066667 0.1 0.133333 0.166667 0.2 0.233333 0.266667 0.3 0.333333 0.366667 0.4 0.433333 0.466667 0.5 0.533333 0.566667 0.6 0.633333 0.666667 0.7 0.733333 0.766667 0.8 0.833333 0.866667 0.9 0.933333 0.966667 0.987061 0.987061 0.987061 0.987061 0.987061 0.987061
  line L0 (1.5, 99.6882) -> (1.5, 49)
  line L1 (1.5, 49) -> (-1.5, 49)
  line L2 (-1.5, 49) -> (-1.5, 99.6882)
  spline S1 degree 5 poles (-1.5, 99.6882) (-1.9488, 99.5793) (-3.0815, 99.2699) (-4.7065, 98.6714) (-6.4983, 97.6092) (-8.0745, 95.7609) (-9.1121, 93.07) (-9.6963, 89.6745) (-10.0586, 85.6893) (-10.424, 81.4506) (-10.99, 77.4724) (-11.907, 74.2934) (-13.2584, 72.3576) (-15.0394, 71.8776) (-17.1367, 72.7086) (-19.3037, 74.2023) (-21.2553, 75.4915) (-22.7671, 75.7922) (-23.7735, 74.6973) (-24.4682, 72.4808) (-25.1834, 69.8088) (-26.2619, 67.4376) (-27.9429, 65.9395) (-30.2155, 65.3602) (-32.8779, 65.334) (-35.6446, 65.308) (-38.2344, 64.7235) (-40.4714, 63.2243) (-42.3664, 60.8266) (-44.0522, 57.789) (-45.7311, 54.5085) (-47.2407, 52.0292) (-48.5446, 50.4053) (-49.5004, 49.4476) (-50, 49) knots -0.987061 -0.987061 -0.987061 -0.987061 -0.987061 -0.987061 -0.966667 -0.933333 -0.9 -0.866667 -0.833333 -0.8 -0.766667 -0.733333 -0.7 -0.666667 -0.633333 -0.6 -0.566667 -0.533333 -0.5 -0.466667 -0.433333 -0.4 -0.366667 -0.333333 -0.3 -0.266667 -0.233333 -0.2 -0.166667 -0.133333 -0.1 -0.066667 -0.033333 0 0 0 0 0 0
  line L3 (-50, 49) -> (-50, 0)
  line L4 (-50, 0) -> (50, 0)
  line L5 (50, 0) -> (50, 49)
equation "d10 = ( 100 / 2 ) * 1 mm"
equation "d12 = ( 3 / 2 ) * 1 mm"

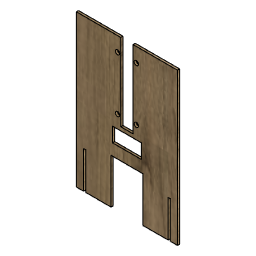
design "WaterLevelSensorHolder"
Autodesk Fusion 360 part; units mm, degrees
sketch "Sketch1" plane through (0, 0, 0) normal (0, 1, 0) x (1, 0, 0)
  line L0 (0, -150) -> (0, 0) construction
  line L1 (-22, 0) -> (-22, -62)
  line L2 (-70, 0) -> (-70, -210)
  line L3 (-75, 0) -> (45, 0) construction
  line L4 (-22, -62) -> (0, -62)
  line L5 (-70, 0) -> (0, 0)
  line L6 (-70, -210) -> (0, -210)
  line L7 (-60, 0) -> (-60, -51)
  line L8 (-57, 0) -> (-57, -51)
  line L9 (-60, -51) -> (-57, -51)
  line L10 (60, 0) -> (60, -51)
  line L11 (60, -51) -> (57, -51)
  line L12 (57, 0) -> (57, -51)
  line L13 (22, 0) -> (22, -62)
  line L14 (70, 0) -> (70, -210)
  line L15 (70, 0) -> (0, 0)
  line L16 (22, -62) -> (0, -62)
  line L17 (70, -210) -> (0, -210)
  dimension "d1" = 22
  dimension "d2" = 70
  dimension "d3" = 62
  dimension "d4" = 210
  dimension "d9" = 51
  dimension "d10" = 10
  dimension "d11" = 51
  dimension "d12" = 3
  constraint coincident L0.end L5.end
  constraint vertical L0
  constraint vertical L1
  constraint parallel L0 L2
  constraint horizontal L3
  constraint coincident L0 L4.end
  constraint perpendicular L0 L4
  constraint perpendicular L2 L5
  constraint coincident L0 L6.end
  constraint perpendicular L0 L6
  constraint coincident L3 L7.start
  constraint coincident L5 L7.start
  constraint perpendicular L5 L7
  constraint coincident L5 L8.start
  constraint perpendicular L5 L8
  constraint symmetric L0 L1.start L13.start
  constraint symmetric L0 L1.end L13.end
  constraint symmetric L0 L2.start L14.start
  constraint symmetric L0 L2.end L14.end
  constraint symmetric L0 L4.end L16.end
  constraint symmetric L0 L5.end L15.end
  constraint symmetric L0 L6.end L17.end
  constraint symmetric L0 L7.start L10.start
  constraint symmetric L0 L7.end L10.end
  constraint symmetric L0 L8.start L12.start
  constraint symmetric L0 L8.end L11.end
  measures "d1" distance of L0 L1
  measures "d2" distance of L0 L2
  measures "d3" distance of L1.start L1.end
  measures "d4" distance of L2.start L2.end
  measures "d9" distance of L7.start L7.end
  measures "d10" distance of L2 L7
  measures "d11" distance of L8.start L8.end
  measures "d12" distance of L7 L8
extrude "Extrude1" add sketch "Sketch1" along normal blind 3 contours L1 L2 L4 L5 L6 L7 L8 L9 L10 L11 L12 L13 L14 L15 L16 L17
sketch "Sketch2" plane through (0, 0, 0) normal (0, 1, 0) x (1, 0, 0)
  line L0 (-13, -190) -> (13, -190) construction
  line L1 (13, -190) -> (13, -116) construction
  line L2 (13, -116) -> (-13, -116) construction
  line L3 (-13, -116) -> (-13, -190) construction
  line L4 (0, -150) -> (0, 0)
  line L5 (-70, -210) -> (0, -210)
  circle A0 centre (-13, -190) radius 3
  circle A1 centre (13, -190) radius 3
  circle A2 centre (-13, -116) radius 3
  circle A3 centre (13, -116) radius 3
  line L6 (-8.5, -210) -> (-8.5, -103)
  line L7 (-8.5, -103) -> (0, -103)
  line L8 (8.5, -210) -> (8.5, -103)
  line L9 (8.5, -103) -> (0, -103)
  line L10 (0, -210) -> (-8.5, -210)
  line L11 (0, -210) -> (8.5, -210)
  line L12 (0, -98) -> (-20, -98)
  line L13 (0, -78) -> (-20, -78)
  line L14 (-20, -98) -> (-20, -78)
  line L15 (0, -98) -> (20, -98)
  line L16 (20, -98) -> (20, -78)
  line L17 (0, -78) -> (20, -78)
  dimension "d15" = 74
  dimension "d16" = 26
  dimension "d17" = 13
  dimension "d18" = 20
  dimension "d19" = 6
  dimension "d20" = 6
  dimension "d21" = 6
  dimension "d22" = 6
  dimension "d26" = 8.5
  dimension "d27" = 107
  dimension "d30" = 5
  dimension "d31" = 20
  dimension "d32" = 20
  dimension "d33" = 20
  constraint horizontal L0
  constraint vertical L1
  constraint horizontal L2
  constraint vertical L3
  constraint coincident L0.start L3.end
  constraint coincident L0.end L1.start
  constraint coincident L2.end L3.start
  constraint coincident L1.end L2.start
  constraint coincident L5 L6.start
  constraint perpendicular L5 L6
  constraint coincident L4 L7.end
  constraint perpendicular L4 L7
  constraint symmetric L4 L6.start L8.start
  constraint symmetric L4 L6.end L8.end
  constraint symmetric L4 L7.end L9.end
  constraint coincident L5.end L10.start
  constraint symmetric L4 L5.end L10.start
  constraint coincident L4 L12.start
  constraint perpendicular L4 L12
  constraint coincident L4 L13.start
  constraint perpendicular L4 L13
  constraint symmetric L4 L12.start L15.start
  constraint symmetric L4 L12.end L15.end
  constraint symmetric L4 L13.start L17.start
  constraint symmetric L4 L13.end L16.end
  measures "d15" distance of L0.end L1.end
  measures "d16" distance of L0.start L0.end
  measures "d17" distance of L3 L4
  measures "d18" distance of L0 L5
  measures "d19" diameter of A0
  measures "d20" diameter of A1
  measures "d21" diameter of A2
  measures "d22" diameter of A3
  measures "d26" distance of L4 L6
  measures "d27" distance of L6.start L6.end
  measures "d30" distance of L7 L12
  measures "d31" distance of L12.start L12.end
  measures "d32" distance of L13.start L13.end
  measures "d33" distance of L12 L13
extrude "Extrude3" cut sketch "Sketch2" along normal blind 3
ref_plane "WorkPlane1" through (0, 0, 105) normal (0, 1, 0) x (1, 0, 0)
sketch "LaserCut" plane through (0, 0, 0) normal (0, 1, 0) x (1, 0, 0)
  line L0 (-8.5, -103) -> (-8.5, -210)
  line L1 (-8.5, -210) -> (-70, -210)
  line L2 (-70, -210) -> (-70, 0)
  line L3 (-70, 0) -> (-60, 0)
  line L4 (-60, 0) -> (-60, -51)
  line L5 (-60, -51) -> (-57, -51)
  line L6 (-57, -51) -> (-57, 0)
  line L7 (-57, 0) -> (-22, 0)
  line L8 (-22, 0) -> (-22, -62)
  line L9 (-22, -62) -> (22, -62)
  line L10 (22, -62) -> (22, 0)
  line L11 (22, 0) -> (57, 0)
  line L12 (57, 0) -> (57, -51)
  line L13 (57, -51) -> (60, -51)
  line L14 (60, -51) -> (60, 0)
  line L15 (60, 0) -> (70, 0)
  line L16 (70, 0) -> (70, -210)
  line L17 (70, -210) -> (8.5, -210)
  line L18 (8.5, -210) -> (8.5, -103)
  line L19 (8.5, -103) -> (-8.5, -103)
  circle A0 centre (-13, -116) radius 3
  circle A1 centre (13, -116) radius 3
  circle A2 centre (13, -190) radius 3
  circle A3 centre (-13, -190) radius 3
  line L20 (-20, -78) -> (-20, -98)
  line L21 (-20, -98) -> (20, -98)
  line L22 (20, -98) -> (20, -78)
  line L23 (20, -78) -> (-20, -78)
equation "d1 = ( 44 / 2 ) * 1 mm"
equation "d17 = ( 26 / 2 ) * 1 mm"

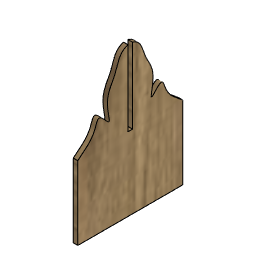
design "Base_Foot_WaterLEvelSensorHolder"
Autodesk Fusion 360 part; units mm, degrees
sketch "Sketch1" plane through (0, 0, 0) normal (1, 0, 0) x (0, 1, 0)
  line L0 (0, 0) -> (0, 100) construction
  spline S0 degree 5 poles (-35, 49.4017) (-34.5671, 49.7896) (-33.6897, 50.5546) (-32.3391, 51.6696) (-30.4956, 53.1165) (-28.2652, 54.9855) (-26.2784, 57.0434) (-24.6758, 59.3564) (-23.5164, 61.869) (-22.719, 64.3332) (-22.0218, 66.2667) (-21.1315, 67.1936) (-19.8358, 66.8284) (-18.1658, 65.3445) (-16.4091, 63.3865) (-14.9295, 61.7511) (-14.0473, 61.1728) (-13.8699, 62.0243) (-14.2266, 64.192) (-14.8056, 67.2875) (-15.2521, 70.7939) (-15.2712, 74.2227) (-14.7555, 77.3008) (-13.7866, 79.9925) (-12.5455, 82.3999) (-11.2515, 84.7018) (-10.0863, 87.0739) (-9.133, 89.625) (-8.2877, 92.3076) (-7.2959, 94.944) (-5.8354, 97.2946) (-4.0331, 98.7486) (-2.2118, 99.5116) (-0.7745, 99.8634) (0, 100) knots 0 0 0 0 0 0 0.033333 0.066667 0.1 0.133333 0.166667 0.2 0.233333 0.266667 0.3 0.333333 0.366667 0.4 0.433333 0.466667 0.5 0.533333 0.566667 0.6 0.633333 0.666667 0.7 0.733333 0.766667 0.8 0.833333 0.866667 0.9 0.933333 0.966667 1 1 1 1 1 1
  spline S1 degree 5 poles (35, 49.4017) (34.5671, 49.7896) (33.6897, 50.5546) (32.3391, 51.6696) (30.4956, 53.1165) (28.2652, 54.9855) (26.2784, 57.0434) (24.6758, 59.3564) (23.5164, 61.869) (22.719, 64.3332) (22.0218, 66.2667) (21.1315, 67.1936) (19.8358, 66.8284) (18.1658, 65.3445) (16.4091, 63.3865) (14.9295, 61.7511) (14.0473, 61.1728) (13.8699, 62.0243) (14.2266, 64.192) (14.8056, 67.2875) (15.2521, 70.7939) (15.2712, 74.2227) (14.7555, 77.3008) (13.7866, 79.9925) (12.5455, 82.3999) (11.2515, 84.7018) (10.0863, 87.0739) (9.133, 89.625) (8.2877, 92.3076) (7.2959, 94.944) (5.8354, 97.2946) (4.0331, 98.7486) (2.2118, 99.5116) (0.7745, 99.8634) (0, 100) knots 0 0 0 0 0 0 0.033333 0.066667 0.1 0.133333 0.166667 0.2 0.233333 0.266667 0.3 0.333333 0.366667 0.4 0.433333 0.466667 0.5 0.533333 0.566667 0.6 0.633333 0.666667 0.7 0.733333 0.766667 0.8 0.833333 0.866667 0.9 0.933333 0.966667 1 1 1 1 1 1
  line L1 (-43.5461, 41.744) -> (-26.4539, 57.0594)
  line L2 (-14.0459, 97.5218) -> (14.0459, 102.4782)
  line L3 (43.5461, 41.744) -> (26.4539, 57.0594)
  line L4 (14.0459, 97.5218) -> (-14.0459, 102.4782)
  line L5 (-75, 100) -> (80, 100) construction
  line L6 (-35, 49.4017) -> (-35, 0.4017)
  line L7 (35, 49.4017) -> (35, 0.4017)
  line L8 (-35, 0.4017) -> (35, 0.4017)
  line L9 (-35, 49.4017) -> (35, 49.4017) construction
  line L10 (-1.5, 49.4017) -> (-1.5, 99.6524)
  line L11 (1.5, 49.4017) -> (1.5, 99.6524)
  line L12 (1.5, 49.4017) -> (-1.5, 49.4017)
  point P0 (-23.7312, 61.5494)
  point P1 (-20.3639, 66.8408)
  point P2 (-14.4311, 61.5494)
  point P3 (-15.2004, 72.2084)
  point P4 (-9.8431, 87.8254)
  point P5 (9.8431, 87.8254)
  point P6 (23.7312, 61.5494)
  point P7 (20.3639, 66.8408)
  point P8 (14.4311, 61.5494)
  point P9 (15.2004, 72.2084)
  dimension "d8" = 100
  dimension "d10" = 35
  dimension "d11" = 49
  dimension "d12" = 1.5
  constraint coincident L0.start origin
  constraint midpoint L1 S0.start
  constraint midpoint L0.end L2
  constraint symmetric L0 S1.start S0.start
  constraint symmetric S0.end L0 S1.end
  constraint symmetric L0 P0 P6
  constraint symmetric L0 P1 P7
  constraint symmetric L0 P2 P8
  constraint symmetric L0 P3 P9
  constraint symmetric L0 P4 P5
  constraint symmetric L0 L1.start L3.start
  constraint symmetric L0 L1.end L3.end
  constraint symmetric L0 L2.start L4.start
  constraint symmetric L0 L2.end L4.end
  constraint horizontal L5
  constraint vertical L6
  constraint symmetric L0 S0.start S1.start
  constraint symmetric L0 L6.end L7.end
  constraint vertical L10
  constraint coincident S0 L10.end
  constraint symmetric L0 L10.start L11.start
  constraint symmetric L0 L10.end L11.end
  constraint coincident L9 L10.start
  measures "d8" distance of L0.start L0.end
  measures "d10" distance of L0 L6
  measures "d11" distance of L8 L9
  measures "d12" distance of L0 L10
extrude "Extrude2" add sketch "Sketch1" along normal blind 3 contours S0 S1 L6 L7 L8 L10 L11 L12
ref_plane "WorkPlane1" through (3, 0, 50.0271) normal (1, 0, 0) x (0, 1, 0)